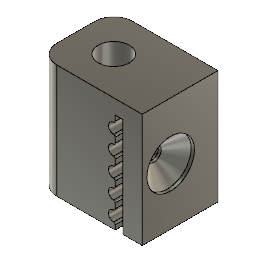
1-All_Belt_Clamps_V2_Clamp_3 (Autodesk Fusion 360 design; units mm, degrees)
Autodesk Fusion 360 part; units mm, degrees
note: some values were not read from the file. Set by a fixed rule: which sketch regions a step uses.
sketch "Bottom Profile" plane through (0, 0, 0) normal (0, 0, 1) x (1, 0, 0)
  line L0 (-4, 4) -> (7, 4)
  line L1 (7, 4) -> (7, -4)
  line L2 (7, -4) -> (-4, -4)
  line L3 (-4, -4) -> (-4, 4)
  circle A0 centre (0, 0) radius 1.625
  line L4 (-4, 0) -> (7, 0) construction
  circle A1 centre (0, 0) radius 3
  dimension "d1" = 11
  dimension "d2" = 8
  dimension "d3" = 3.25
  dimension "d4" = 4
  dimension "d5" = 6
  constraint horizontal L0
  constraint vertical L1
  constraint horizontal L2
  constraint vertical L3
  constraint coincident A0.centre A1.centre
  constraint midpoint L3 L4.start
  constraint midpoint L1 L4.end
  constraint coincident A0.centre L4
  measures "d1" distance of L0.start L0.end
  measures "d2" distance of L0.start L2.end
  measures "d3" diameter of A0
  measures "d4" distance of L3 A0.centre
  measures "d5" diameter of A1
extrude "Extrude1" add sketch "Bottom Profile" along normal blind 12 contours L0 L1 L2 L3 | A1
extrude "Extrude2" cut sketch "Bottom Profile" along normal blind 2 contours A1
sketch "Trapezoidal Cutout" plane through (-4, 0, 0) normal (-1, 0, 0) x (0, -1, 0)
  line L0 (-4, 0) -> (4, 0)
  line L1 (4, 0) -> (4, 12)
  line L2 (4, 12) -> (-4, 12)
  line L3 (-4, 12) -> (-4, 0)
  line L4 (-2, 1) -> (2, 1)
  line L5 (2, 1) -> (3, 0)
  line L6 (-2, 1) -> (-3, 0)
  line L7 (0, 0) -> (0, 1) construction
  line L8 (4, 0) -> (-4, 0)
  dimension "d10" = 1
  dimension "d11" = 135
  dimension "d12" = 135
  dimension "d13" = 4
  constraint perpendicular L3 L4
  constraint coincident L0 L5.end
  constraint coincident L0 L6.end
  constraint coincident L7.start origin
  constraint midpoint L4 L7.end
  constraint vertical L7
  measures "d10" distance of L4 L8
  measures "d11" angle of L4 L6
  measures "d12" angle of L4 L5
  measures "d13" distance of L4.start L4.end
extrude "Extrude3" cut sketch "Trapezoidal Cutout" along normal up to surface contours L0 L4 L5 L6 L8 end surface at (2.9963, -0.1495, 1.3333)
sketch "Cross Hole" plane through (7, 0, 0) normal (1, 0, 0) x (0, 1, 0)
  line L0 (-4, 0) -> (4, 0)
  line L1 (4, 0) -> (4, 12)
  line L2 (4, 12) -> (-4, 12)
  line L3 (-4, 12) -> (-4, 0)
  circle A0 centre (-1, 6) radius 0.75
  circle A1 centre (-1, 6) radius 2.5
  dimension "d16" = 1.5
  dimension "d17" = 5
  dimension "d18" = 3
  dimension "d19" = 6
  constraint concentric A0 A1
  measures "d16" diameter of A0
  measures "d17" diameter of A1
  measures "d18" distance of L3 A0.centre
  measures "d19" distance of L0 A0.centre
extrude "Extrude4" cut sketch "Cross Hole" against normal blind 9 contours A0
extrude "Extrude5" cut sketch "Cross Hole" against normal blind 1.75 contours A1
chamfer "Chamfer1" distance 1.4 distance2 1.75 1 edges at (5.25, -3.3308, 6.904) measured on face at (5.8333, 1.4876, 5.7511)
sketch "Belt Profile" plane through (0, -4, 0) normal (0, -1, 0) x (1, 0, 0)
  line L0 (-4, 0) -> (7, 0)
  line L1 (7, 0) -> (7, 12)
  line L2 (7, 12) -> (-4, 12)
  line L3 (-4, 12) -> (-4, 0)
  line L4 (4.15, 10.5) -> (4.95, 10.5)
  line L5 (4.95, 10.5) -> (4.95, 0)
  line L6 (4.95, 0) -> (4.15, 0)
  line L7 (4.15, 0) -> (4.15, 10.5)
  circle A0 centre (3.99, 1.21) radius 0.55
  line L8 (3.99, 1.76) -> (4.15, 1.76)
  line L9 (3.99, 0.66) -> (4.15, 0.66)
  circle A1 centre (3.99, 3.21) radius 0.55
  line L10 (3.99, 2.66) -> (4.15, 2.66)
  line L11 (3.99, 3.76) -> (4.15, 3.76)
  circle A2 centre (3.99, 5.21) radius 0.55
  line L12 (3.99, 4.66) -> (4.15, 4.66)
  line L13 (3.99, 5.76) -> (4.15, 5.76)
  circle A3 centre (3.99, 7.21) radius 0.55
  line L14 (3.99, 6.66) -> (4.15, 6.66)
  line L15 (3.99, 7.76) -> (4.15, 7.76)
  circle A4 centre (3.99, 9.21) radius 0.55
  line L16 (3.99, 8.66) -> (4.15, 8.66)
  line L17 (3.99, 9.76) -> (4.15, 9.76)
  dimension "d26" = 2.05
  dimension "d27" = 0.8
  dimension "d28" = 1.1
  dimension "d29" = 1.21
  dimension "d30" = 0.16
  dimension "d33" = 2
  dimension "d34" = 0
  dimension "d35" = 10.5
  constraint horizontal L4
  constraint vertical L5
  constraint horizontal L6
  constraint vertical L7
  constraint coincident L0 L5.end
  constraint coincident A0 L8.start
  constraint tangent A0 L8
  constraint coincident L7 L8.end
  constraint perpendicular L7 L8
  constraint coincident A0 L9.start
  constraint tangent A0 L9
  constraint coincident L7 L9.end
  constraint perpendicular L7 L9
  measures "d26" distance of L1 L5
  measures "d27" distance of L5 L7
  measures "d28" diameter of A0
  measures "d29" distance of L0 A0.centre
  measures "d30" horizontal distance of L6.end A0.centre
  measures "d35" distance of L0 L4
extrude "Extrude6" cut sketch "Belt Profile" against normal blind 6.1 contours L0 L4 L5 L6 L7 A0 A1 A2 A3 A4 | L7 A0 L9 | L7 A0 | L7 A0 | L7 A0 L8 | L7 A4 L17 | L7 A4 | L7 A4 | L7 A1 L10 | L7 A4 L16 | L7 A1 | L7 A1 | L7 A1 L11 | L7 A3 L15 | L7 A3 | L7 A3 | L7 A2 L12 | L7 A3 L14 | L7 A2 | L7 A2 | L7 A2 L13
fillet "Fillet2" radius 0.175 12 edges at (4.15, -0.95, 1.76) (4.15, -0.95, 2.66) (4.15, -0.95, 3.76) (4.15, -0.95, 4.66) (4.15, -2.6781, 6.66) (4.15, -2.8553, 5.76) (4.15, -0.95, 8.66) (4.15, -0.95, 7.76) (4.15, -0.95, 9.76) (4.15, 0.7281, 6.66) (4.15, 0.9053, 5.76) (4.15, -0.95, 0.66)
fillet "Fillet1" radius 2 2 edges at (-4, -4, 6) (-4, 4, 6)
named bodies: "1-All_Belt_Clamps V2 Clamp 3"
